Bielle 2 (Autodesk Fusion 360 design; units mm, degrees)
Autodesk Fusion 360 part; units mm, degrees
note: some values were not read from the file. Chosen so that the rebuilt part matches the saved one: which face or edge a step refers to. Set by a fixed rule: which sketch regions a step uses.
sketch "Sketch1" plane through (0, 0, 0) normal (0, 0, 1) x (1, 0, 0)
  circle A0 centre (0, 0) radius 16.75
  dimension "d1" = 33.5
  constraint coincident A0.centre origin
  measures "d1" diameter of A0
extrude "Extrude1" add sketch "Sketch1" along normal blind 11 makes body 1
sketch "Sketch2" plane through (0, 0, 11) normal (0, 0, 1) x (-1, 0, 0)
  circle A0 centre (0, 0) radius 16.75
  circle A1 centre (0, 0) radius 21.5
  dimension "d4" = 43
  constraint coincident A0.centre A1.centre
  measures "d4" diameter of A1
extrude "Extrude2" add sketch "Sketch2" along normal blind 5 contours A0 | A1 bodies 1
chamfer "Chamfer1" distance 2 distance2 5 1 edges at (20.045, 7.7747, 16) measured on face at (0.08, -1.0681, 16) on bodies 1
sketch "Sketch3" plane through (0, 0, 16) normal (0, 0, 1) x (-1, 0, 0)
  circle A0 centre (0, 0) radius 19.5
  circle A1 centre (0, 0) radius 15
  dimension "d10" = 30
  constraint coincident A0.centre A1.centre
  measures "d10" diameter of A1
extrude "Extrude3" add sketch "Sketch3" along normal blind 17 contours A1 bodies 1
ref_plane "WorkPlane1" through (12.125, 0, 0) normal (0, 0.207912, 0.978148) x (1, 0, 0)
ref_plane "WorkPlane2" through (12.125, 4.5117, 21.2258) normal (0, 0.207912, 0.978148) x (1, 0, 0)
split "Split1" by plane through (12.125, 4.5117, 21.2258) normal (0, 0.207912, 0.978148) bodies 1 makes body 2 at (-2.338, 14.8167, 28.3475)
extrude "Extrude4" add 1 faces at (4.9784, 0.274, 22.1265) along direction (0, 0.207912, 0.978148) blind 35 on bodies 1 bodies 1
sketch "Sketch7" plane through (0, 0, 0) normal (0, 0, -1) x (1, 0, 0)
  circle A0 centre (0, 0) radius 16.75
  circle A1 centre (0, 0) radius 5.25
  dimension "d33" = 10.5
  constraint coincident A0.centre A1.centre
  measures "d33" diameter of A1
extrude "Extrude9" cut sketch "Sketch7" against normal through all contours A1 bodies 1
ref_plane "WorkPlane3" through (0, 0, 62) normal (0, 0, 1) x (1, 0, 0)
sketch "Sketch8" plane through (0, 0, 62) normal (0, 0, 1) x (1, 0, 0)
  circle A0 centre (0, 0) radius 11.1
  dimension "d36" = 22.2
  constraint coincident A0.centre origin
  measures "d36" diameter of A0
extrude "Extrude10" cut sketch "Sketch8" against normal blind 28 bodies 1
ref_plane "WorkPlane4" through (0, 0, 11) normal (0, 0, -1) x (1, 0, 0)
split "Split2" by plane through (0, 0, 11) normal (0, 0, -1) bodies 1 makes body 3 at (16.7292, -0.8349, 7.3333)
sketch "Sketch9" plane through (0, 0, 11) normal (0, 0, -1) x (1, 0, 0)
  circle A0 centre (0, 0) radius 4.5
  circle A1 centre (0, 0) radius 16.75
  line L0 (10.1, 5.8312) -> (0, 11.6625)
  line L1 (0, 11.6625) -> (-10.1, 5.8312)
  line L2 (-10.1, 5.8312) -> (-10.1, -5.8312)
  line L3 (-10.1, -5.8312) -> (0, -11.6625)
  line L4 (0, -11.6625) -> (10.1, -5.8312)
  line L5 (10.1, -5.8312) -> (10.1, 5.8312)
  circle A2 centre (0, 0) radius 21.5
  circle A3 centre (0, 0) radius 5.25
  dimension "d51" = 10.1
  constraint coincident A0.centre A1.centre
  measures "d51" distance of A0.centre L5
ref_plane "WorkPlane6" through (0, 2.99, 36.2518) normal (0, -0.978148, 0.207912) x (0, 0.207912, 0.978148)
ref_plane "WorkPlane7" through (0, 12.7715, 34.1727) normal (0, -0.978148, 0.207912) x (0, 0.207912, 0.978148)
sketch "Sketch10" plane through (0, 12.7715, 34.1727) normal (0, -0.978148, 0.207912) x (0, 0.207912, 0.978148)
  line L0 (20.6187, -15) -> (20.6187, 15)
  line L1 (-14.3813, -15) -> (-14.3813, 15)
  line L2 (-14.3813, -15) -> (-14.3813, 15)
  line L3 (20.6187, 15) -> (-14.3813, -15) construction
  line L4 (20.6187, 0) -> (-14.3813, 0) construction
  line L5 (20.6187, -2.5) -> (-14.3813, -2.5)
  line L6 (-14.3813, -2.5) -> (-14.3813, 2.5)
  line L7 (-14.3813, 2.5) -> (20.6187, 2.5)
  line L8 (20.6187, 2.5) -> (20.6187, -2.5)
  dimension "d58" = 5
  constraint coincident L0.end L3.start
  constraint coincident L1.start L2.start
  constraint midpoint L0 L4.start
  constraint midpoint L2 L4.end
  constraint horizontal L5
  constraint vertical L6
  constraint horizontal L7
  constraint vertical L8
  constraint coincident L1 L6.end
  constraint coincident L0 L5.start
  constraint midpoint L4.start L8
  measures "d58" distance of L5.start L7.end
extrude "Extrude14" add sketch "Sketch10" against normal blind 7 bodies 1
extrude "Extrude11" cut sketch "Sketch9" against normal blind 11 contours L0 L1 L2 L3 L4 L5 bodies 1
extrude "Extrude17" cut 1 faces at (0.8333, 21.4798, 41.4737) along direction (0, -0.978148, 0.207912) blind 5 on bodies 1 bodies 1
extrude "Extrude18" add 1 faces at (0.2789, 12.8174, 19.4604) along direction (0, 0.207912, 0.978148) blind 3 on bodies 1 bodies 1
sketch "Sketch12" plane through (0, 0, 34) normal (0, 0, 1) x (-1, 0, 0)
  circle A0 centre (0, 0) radius 5.25
  circle A1 centre (0, 0) radius 11.1
  circle A2 centre (0, 0) radius 6.5
  dimension "d73" = 13
  constraint coincident A0.centre A1.centre
  measures "d73" diameter of A2
extrude "Extrude19" [suppressed]
hidden bodies 2 3
